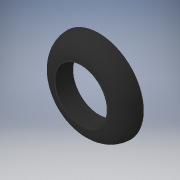
# Autodesk Inventor part: Part7
Saved by Autodesk Inventor 2019 (Build 230136000, 136)
## iProperties
Created: 2019-08-22
Part Number: Part7
Material: Rubber
Document SubType Name: Modeling
Designer: bowen.wu2
Density: 0.93 g/cm^3
Appearance: Rubber - Black
Author: bowen.wu2
Autodesk Inventor part; units mm, degrees
ref_plane "YZ Plane" through (0, 0, 0) normal (1, 0, 0) x (0, 1, 0)
ref_plane "XZ Plane" through (0, 0, 0) normal (0, 1, 0) x (-1, 0, 0)
ref_plane "XY Plane" through (0, 0, 0) normal (0, 0, 1) x (1, 0, 0)
sketch "Sketch1" plane through (0, 0, 0) normal (0, 0, 1) x (1, 0, 0)
  circle A0 centre (0, 0) radius 1.45
  circle A1 centre (0, 0) radius 2.5
  dimension "d0" = 2.9
  dimension "d1" = 5
  constraints: 2 centre point, 2 coincident
  measures "d0" diameter of A0
  measures "d1" diameter of A1
extrude "Extrusion1" add sketch "Sketch1" along normal blind 1
fillet "Fillet1" radius 1 1 edges at (-2.5, 0, 1)
body "Solid1"
